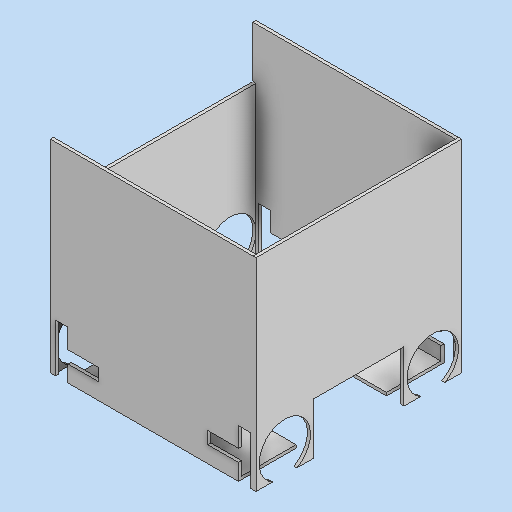
# Autodesk Inventor part: Chassis Conceptual Geo
Saved by Autodesk Inventor 2026 (Build 300175000, 175)
## iProperties
Created: 2026-01-28
Part Number: Chassis Conceptual Geo
Material: Generic
Document SubType Name: Modeling
Designer: mones
Density: 1 g/cm^3
Appearance: Default
Author: mones
Autodesk Inventor part; units mm, degrees
ref_plane "YZ Plane" through (0, 0, 0) normal (1, 0, 0) x (0, 1, 0)
ref_plane "XZ Plane" through (0, 0, 0) normal (0, 1, 0) x (-1, 0, 0)
ref_plane "XY Plane" through (0, 0, 0) normal (0, 0, 1) x (1, 0, 0)
sketch "Sketch1" plane through (0, 0, 0) normal (0, 0, 1) x (1, 0, 0)
  line L0 (-200.0185, 197.9846) -> (-0.0185, -2.0154) construction
  line L1 (-200.0185, -2.0154) -> (-0.0185, 197.9846) construction
  line L2 (-200.0185, 2.9846) -> (-0.0185, 2.9846)
  line L3 (-0.0185, 2.9846) -> (-5.0185, 2.9846)
  line L4 (-17.0185, -0.0154) -> (-5.0185, -0.0154)
  line L5 (-17.0185, 6.9846) -> (-17.0185, 18.9846)
  line L6 (-47.0185, 6.9846) -> (-17.0185, 18.9846) construction
  line L7 (-17.0185, 6.9846) -> (-47.0185, 18.9846) construction
  line L8 (-195.0185, 25.9846) -> (-195.0185, -0.0154)
  line L9 (-195.0185, -0.0154) -> (-183.0185, -0.0154)
  line L10 (-183.0185, -0.0154) -> (-183.0185, 25.9846)
  line L11 (-183.0185, 25.9846) -> (-195.0185, -0.0154) construction
  line L12 (-195.0185, 25.9846) -> (-183.0185, -0.0154) construction
  line L13 (-168.0185, 12.9846) -> (-183.0185, 6.9846) construction
  line L14 (-0.0185, 2.9846) -> (-0.0185, 199.9846)
  line L15 (-0.0185, 199.9846) -> (-200.0185, 199.9846)
  line L16 (-200.0185, 2.9846) -> (-200.0185, 199.9846)
  line L17 (-183.0185, 18.9846) -> (-180.1613, 17.8418) construction
  line L18 (-168.0185, 12.9846) -> (-153.0185, 6.9846) construction
  line L19 (-5.0185, 0) -> (-17.0185, 0)
  line L20 (-183.0185, 0) -> (-195.0185, 0)
  line L21 (-5.0185, 0) -> (-5.0185, 50)
  line L22 (-17.0185, 0) -> (-17.0185, 50)
  line L23 (-17.0185, 50) -> (-5.0185, 50)
  line L24 (-5.0185, 25) -> (-47.0185, 25)
  line L25 (-47.0185, 19) -> (-5.0185, 19)
  line L26 (-5.0185, 19) -> (-5.0185, 31)
  line L27 (-5.0185, 31) -> (-47.0185, 31)
  line L28 (-47.0185, 31) -> (-47.0185, 19)
  line L29 (-47.0185, 19) -> (-5.0185, 31) construction
  line L30 (-5.0185, 19) -> (-47.0185, 31) construction
  line L31 (-183.0185, 0) -> (-183.0185, 50)
  line L32 (-195.0185, 0) -> (-195.0185, 50)
  line L33 (-195.0185, 50) -> (-183.0185, 50)
  line L34 (-195.0185, 25) -> (-153.0185, 25)
  line L35 (-153.0185, 19) -> (-195.0185, 19)
  line L36 (-195.0185, 19) -> (-195.0185, 31)
  line L37 (-195.0185, 31) -> (-153.0185, 31)
  line L38 (-153.0185, 31) -> (-153.0185, 19)
  line L39 (-153.0185, 19) -> (-195.0185, 31) construction
  line L40 (-195.0185, 19) -> (-153.0185, 31) construction
  point P0 (-32.0185, 12.9846)
  point P1 (-26.0185, 25)
  point P2 (-174.0185, 25)
  point P3 (-195.0185, 2.9846)
  point P4 (-183.0185, 31)
  point P5 (-183.0185, 19)
  point P6 (-183.0185, 2.9846)
  point P7 (-17.0185, 2.9846)
  point P8 (-17.0185, 19)
  point P9 (-17.0185, 31)
  dimension "d63" = 50
  dimension "d64" = 50
  dimension "d65" = 42
  dimension "d66" = 12
  dimension "d67" = 50
  dimension "d68" = 50
  dimension "d69" = 42
  dimension "d70" = 12
  constraints: 83 end point, 10 midpoint, 8 parallel, 5 point on line, 4 horizontal, 4 perpendicular, 4 vertical
  measures "d63" distance of L19.start L21.end
  measures "d64" distance of L19.end L22.end
  measures "d65" distance of L24.start L24.end
  measures "d66" distance of L26.end L25.end
  measures "d67" distance of L20.start L31.end
  measures "d68" distance of L20.end L32.end
  measures "d69" distance of L34.start L34.end
  measures "d70" distance of L35.end L36.end
sketch "Sketch3" plane through (0, 0, 0) normal (1, 0, 0) x (0, 1, 0)
  line L0 (3, -200) -> (200, -200)
  line L1 (200, -200) -> (200, 0)
  line L2 (200, 0) -> (3, 0)
  line L3 (3, -200) -> (3, -185)
  line L4 (3, 0) -> (3, -30)
  line L5 (3, 0) -> (3, -30)
  line L6 (3, -170) -> (3, -200)
  line L7 (3, -200) -> (3, -144)
  line L8 (3, 0) -> (3, -56)
  line L9 (3, -56) -> (53, -56)
  line L10 (3, -144) -> (53, -144)
  line L11 (53, -144) -> (53, -56)
  line L12 (3, 0) -> (3, -28)
  line L13 (3, -28) -> (25, -28)
  line L14 (3, -172) -> (25, -172)
  circle A0 centre (25, -28) radius 25
  circle A1 centre (25, -172) radius 25
  point P0 (3, -16.1257)
  point P1 (3, -39.8743)
  point P2 (3, -160.1257)
  point P3 (3, -183.8743)
  dimension "d71" = 56
  dimension "d72" = 56
  dimension "d73" = 50
  dimension "d74" = 50
  dimension "d75" = 22
  dimension "d76" = 22
  dimension "d77" = 50
  dimension "d78" = 50
  constraints: 30 end point, 3 horizontal, 3 midpoint, 3 perpendicular, 2 centre point, 2 coincident, 2 point on line, 1 vertical
  measures "d71" distance of L0.start L7.end
  measures "d72" distance of L2.end L8.end
  measures "d73" distance of L8.end L9.end
  measures "d74" distance of L7.end L10.end
  measures "d75" distance of L12.end L13.end
  measures "d76" distance of L14.start L14.end
  measures "d77" diameter of A0
  measures "d78" diameter of A1
extrude "Extrusion1" add sketch "Sketch1" against normal blind 3 contours L21 L23 L22 L27 L28 L25 L5 L2 L10 L35 L38 L37 L31 L33 L32 L8 L16 L15 L14
extrude "Extrusion2" add sketch "Sketch3" against normal blind 3 contours L3 L6 A1 L7 L10 L11 L9 L8 A0 L4 L2 L1 L0
sketch "Sketch4" plane through (-200.0185, 2.9846, 0) normal (-1, 0, 0) x (0, 0, 1)
  line L0 (-3, 197) -> (-3, 22.0154) projected
  line L1 (0, 197) -> (-3, 197) projected
  line L2 (0, 197) -> (0, 197.0154) projected
  line L3 (0, 197.0154) -> (-200, 197.0154) projected
  line L4 (-200, 197.0154) -> (-200, 0.0154) projected
  line L5 (-200, 0.0154) -> (-183.8743, 0.0154) projected
  arc A0 (-160.1257, 0.0154) -> (-183.8743, 0.0154) centre (-172, 22.0154) ccw projected
  line L6 (-160.1257, 0.0154) -> (-144, 0.0154) projected
  line L7 (-144, 0.0154) -> (-144, 50.0154) projected
  line L8 (-144, 50.0154) -> (-56, 50.0154) projected
  line L9 (-56, 50.0154) -> (-56, 0.0154) projected
  line L10 (-56, 0.0154) -> (-39.8743, 0.0154) projected
  arc A1 (-3, 22.0154) -> (-39.8743, 0.0154) centre (-28, 22.0154) ccw projected
  line L11 (-3, 0) -> (-3, 197) projected
  line L12 (-16.1257, 0.0154) -> (-3, 0.0154) projected
  arc A2 (-16.1257, 0.0154) -> (-3, 22.0154) centre (-28, 22.0154) ccw projected
  line L13 (-144, 0.0154) -> (-56, 0.0154)
  line L14 (-200, 197.0154) -> (-200, 147.0154)
  line L15 (-200, 147.0154) -> (-3, 147.0154)
  point P0 (-3, 147.0154)
  dimension "d87" = 50
  constraints: 6 end point, 2 point on line, 1 horizontal, 1 perpendicular
  measures "d87" distance of L3.end L14.end
extrude "Extrusion3" add sketch "Sketch4" against normal blind 3 contours L11 L12 A2 | L0 A1 L10 L9 L8 L7 L6 A0 L5 L4 L15 | L13 L7 L8 L9
sketch "Sketch5" plane through (-200.0185, 3, -200) normal (0, 0, -1) x (-1, 0, 0)
  line L0 (-3, 0) -> (-3, 22) projected
  line L1 (0, 196.9846) -> (-197.0185, 196.9846) projected
  line L2 (-197.0185, 196.9846) -> (-197.0185, 22) projected
  line L3 (-197.0185, 22) -> (-197.0185, 0) projected
  line L4 (-197.0185, 0) -> (-200, 0) projected
  line L5 (-200, 0) -> (-200, -0.0154) projected
  line L6 (-200, -0.0154) -> (-195, -0.0154) projected
  line L7 (-195, -0.0154) -> (-195, 47) projected
  line L8 (-195, 47) -> (-183, 47) projected
  line L9 (-183, 47) -> (-183, 28) projected
  line L10 (-183, 28) -> (-153, 28) projected
  line L11 (-153, 28) -> (-153, 16) projected
  line L12 (-153, 16) -> (-183, 16) projected
  line L13 (-183, 16) -> (-183, -0.0154) projected
  line L14 (-183, -0.0154) -> (-17, -0.0154) projected
  line L15 (-17, -0.0154) -> (-17, 16) projected
  line L16 (-17, 16) -> (-47, 16) projected
  line L17 (-47, 16) -> (-47, 28) projected
  line L18 (-47, 28) -> (-17, 28) projected
  line L19 (-17, 28) -> (-17, 47) projected
  line L20 (-17, 47) -> (-5, 47) projected
  line L21 (-5, 47) -> (-5, -0.0154) projected
  line L22 (-5, -0.0154) -> (0, -0.0154) projected
  line L23 (0, -0.0154) -> (0, 0) projected
  line L24 (-3, 147) -> (0, 147) projected
  line L25 (0, 147) -> (0, 196.9846) projected
  line L26 (0, 0) -> (-3, 0) projected
  line L27 (-3, 22) -> (-3, 147) projected
extrude "Extrusion4" add sketch "Sketch5" against normal blind 3
sketch "Sketch6" plane through (0, 3, -56) normal (0, -1, 0) x (1, 0, 0)
  line L0 (-3, 53) -> (-0.0185, 53) projected
  line L1 (-3, 39.8743) -> (-3, 53) projected
  line L2 (0, 39.8743) -> (-3, 39.8743) projected
  line L3 (0, 56) -> (0, 39.8743) projected
  line L4 (0, 56) -> (-0.0185, 56) projected
  line L5 (-0.0185, 53) -> (-0.0185, 56) projected
  line L6 (-5.0185, 56) -> (-0.0185, 56) projected
  line L7 (-5.0185, 56) -> (-5.0185, 53) projected
  line L8 (-0.0185, 53) -> (-5.0185, 53) projected
  line L9 (-0.0185, 56) -> (-0.0185, 53) projected
  line L10 (0, 16.1257) -> (0, 0) projected
  line L11 (0, 16.1257) -> (-3, 16.1257) projected
  line L12 (-3, 0) -> (-3, 16.1257) projected
  line L13 (0, 0) -> (-3, 0) projected
  line L14 (0, -88) -> (0, -104.1257) projected
  line L15 (0, -88) -> (-3, -88) projected
  line L16 (-3, -104.1257) -> (-3, -88) projected
  line L17 (0, -104.1257) -> (-3, -104.1257) projected
  line L18 (-0.0185, -141) -> (-0.0185, -144) projected
  line L19 (0, -144) -> (-0.0185, -144) projected
  line L20 (0, -127.8743) -> (0, -144) projected
  line L21 (0, -127.8743) -> (-3, -127.8743) projected
  line L22 (-3, -141) -> (-3, -127.8743) projected
  line L23 (-3, -141) -> (-0.0185, -141) projected
  line L24 (-0.0185, -144) -> (-5.0185, -144) projected
  line L25 (-0.0185, -144) -> (-0.0185, -141) projected
  line L26 (-5.0185, -141) -> (-0.0185, -141) projected
  line L27 (-5.0185, -144) -> (-5.0185, -141) projected
  line L28 (-17.0185, -144) -> (-183.0185, -144) projected
  line L29 (-17.0185, -144) -> (-17.0185, -141) projected
  line L30 (-183.0185, -141) -> (-17.0185, -141) projected
  line L31 (-183.0185, -144) -> (-183.0185, -141) projected
  line L32 (-195.0185, -144) -> (-200.0185, -144) projected
  line L33 (-195.0185, -144) -> (-195.0185, -141) projected
  line L34 (-200.0185, -141) -> (-195.0185, -141) projected
  line L35 (-200.0185, -144) -> (-200.0185, -141) projected
  line L36 (-200.0185, -141) -> (-197.0185, -141) projected
  line L37 (-197.0185, -127.8743) -> (-197.0185, -141) projected
  line L38 (-200.0185, -127.8743) -> (-197.0185, -127.8743) projected
  line L39 (-200.0185, -141) -> (-200.0185, -127.8743) projected
  line L40 (-200.0185, -104.1257) -> (-200.0185, 16.1257) projected
  line L41 (-200.0185, -104.1257) -> (-197.0185, -104.1257) projected
  line L42 (-197.0185, 16.1257) -> (-197.0185, -104.1257) projected
  line L43 (-183.0185, 56) -> (-17.0185, 56) projected
  line L44 (-183.0185, 56) -> (-183.0185, 53) projected
  line L45 (-17.0185, 53) -> (-183.0185, 53) projected
  line L46 (-17.0185, 56) -> (-17.0185, 53) projected
  line L47 (-200.0185, 56) -> (-195.0185, 56) projected
  line L48 (-200.0185, 56) -> (-200.0185, 53) projected
  line L49 (-195.0185, 53) -> (-200.0185, 53) projected
  line L50 (-195.0185, 56) -> (-195.0185, 53) projected
  line L51 (-200.0185, 39.8743) -> (-200.0185, 53) projected
  line L52 (-200.0185, 39.8743) -> (-197.0185, 39.8743) projected
  line L53 (-197.0185, 53) -> (-197.0185, 39.8743) projected
  line L54 (-200.0185, 53) -> (-197.0185, 53) projected
  line L55 (-200.0185, 0) -> (-200.0185, 16.1257) projected
  line L56 (-200.0185, 0) -> (-197.0185, 0) projected
  line L57 (-197.0185, 16.1257) -> (-197.0185, 0) projected
  line L58 (-200.0185, 16.1257) -> (-197.0185, 16.1257) projected
  line L59 (-17.0185, 53) -> (-17.0185, -141)
  line L60 (-3, 0) -> (-197.0185, 0)
  line L61 (-183.0185, 53) -> (-183.0185, -141)
  line L62 (-197.0185, -88) -> (-3, -88)
  line L63 (-200.0185, 16.1257) -> (-197.0185, 16.1257) projected
  line L64 (-197.0185, -88) -> (-157.0185, -88)
  line L65 (-157.0185, -88) -> (-157.0185, 0)
  point P0 (-17.0185, -88)
  point P1 (-183.0185, -88)
  point P2 (-183.0185, 0)
  point P3 (-17.0185, 0)
  dimension "d88" = 40
  constraints: 12 end point, 4 perpendicular, 2 point on line, 1 vertical
  measures "d88" distance of L62.start L64.end
extrude "Extrusion5" add sketch "Sketch6" against normal blind 3 contours L30 L61 L62 L59 | L60 L61 L45 L59
body "Solid1"
